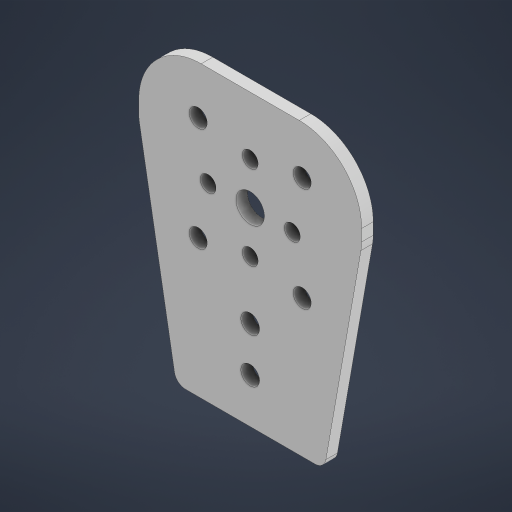
# Autodesk Inventor part: Arm Plate3
Saved by Autodesk Inventor 2024 (Build 280153000, 153)
## iProperties
Created: 2023-10-19
Part Number: Arm Plate3
Material: Generic
Document SubType Name: Modeling
Designer: ellen
Density: 1 g/cm^3
Appearance: Default
Author: ellen
Autodesk Inventor part; units mm, degrees
ref_plane "YZ Plane" through (0, 0, 0) normal (1, 0, 0) x (0, 1, 0)
ref_plane "XZ Plane" through (0, 0, 0) normal (0, 1, 0) x (-1, 0, 0)
ref_plane "XY Plane" through (0, 0, 0) normal (0, 0, 1) x (1, 0, 0)
sketch "Sketch1" plane through (0, 0, 0) normal (0, 0, 1) x (1, 0, 0)
  line L0 (63.5, 76.2) -> (0, 76.2)
  line L1 (0, 76.2) -> (0, 53.975)
  circle A0 centre (31.75, 47.625) radius 4.05
  line L2 (0, 53.975) -> (10.6456, -6.35)
  line L3 (63.5, 53.975) -> (52.8544, -6.35)
  line L4 (10.6456, -6.35) -> (52.8544, -6.35)
  line L5 (63.5, 53.975) -> (63.5, 76.2)
  line L6 (31.75, 76.2) -> (31.75, -6.35)
  circle A1 centre (31.75, 19.05) radius 2.6543
  circle A2 centre (31.75, 6.35) radius 2.6543
  point P0 (0, 0)
  dimension "d0" = 63.5
  dimension "d2" = 8.1
  dimension "d5" = 28.575
  dimension "d50" = 82.55
  dimension "d54" = 5.3086
  dimension "d55" = 57.15
  dimension "d56" = 5.3086
  dimension "d57" = 69.85
  constraints: 14 end point, 3 centre point, 3 point on line, 2 midpoint, 2 parallel, 1 horizontal, 1 perpendicular, 1 vertical
  measures "d0" distance of L0.end L0.start
  measures "d2" diameter of A0
  measures "d5" distance of A0.centre L6.start
  measures "d50" distance between parallel lines of L4 L0
  measures "d54" diameter of A1
  measures "d55" distance from line of L0 A1.centre
  measures "d56" diameter of A2
  measures "d57" distance from line of L0 A2.centre
extrude "Extrusion1" add sketch "Sketch1" along normal blind 3.302 contours L5 L3 L4 L6 A2 A1 A0 L0 | L6 A0 A1 A2 L4 L2 L1 L0
fillet "Fillet9" radius 12.7 1 edges at (63.5, 53.975, 1.651)
fillet "Fillet10" radius 12.7 1 edges at (0, 53.975, 1.651)
fillet "Fillet11" radius 17.78 1 edges at (63.5, 76.2, 1.651)
fillet "Fillet12" radius 17.78 1 edges at (0, 76.2, 1.651)
fillet "Fillet13" radius 3.175 1 edges at (52.8544, -6.35, 1.651)
fillet "Fillet14" radius 3.175 1 edges at (10.6456, -6.35, 1.651)
sketch "Sketch3" plane through (0, 0, 3.302) normal (0, 0, 1) x (1, 0, 0)
  circle A0 centre (31.75, 47.625) radius 4.05 projected
  circle A1 centre (31.75, 47.625) radius 16
  circle A2 centre (31.75, 47.625) radius 8
  circle A3 centre (31.75, 47.625) radius 12
  line L0 (31.75, 47.625) -> (31.75, 69.8383)
  line L1 (31.75, 47.625) -> (53.9633, 47.625) construction
  point P0 (0, 0)
  point P1 (31.75, 59.625)
  dimension "d28" = 24
  dimension "d26" = 32
  dimension "d27" = 16
  dimension "d36" = 90
  constraints: 4 end point, 3 coincident, 2 centre point, 1 horizontal, 1 perpendicular, 1 point on line, 1 vertical alignment, 2 other
  measures "d26" diameter of A1
  measures "d27" diameter of A2
  measures "d36" angle of L1 L0
hole "Hole1" at (31.75, 59.625, 3.302) direction (0, 0, -1) diameter 4.4958 depth 14.1986 tip angle 118 clearance for "Flat Head Machine Screw" size "M4" standard "Ansi Metric M Profile"
pattern_circular "Circular Pattern1" count 4 over 360 about axis through (31.75, 47.625, 0) along (0, 0, 1) of "Hole1"
sketch "Sketch4" plane through (0, 0, 3.302) normal (0, 0, 1) x (1, 0, 0)
  circle A0 centre (31.75, 47.625) radius 4.05 projected
  circle A1 centre (31.75, 47.625) radius 12
  circle A2 centre (31.75, 47.625) radius 16
  circle A3 centre (31.75, 47.625) radius 20.955
  line L0 (45.72, 76.2) -> (17.78, 76.2) projected
  line L1 (31.75, 47.625) -> (51.1677, 67.0427)
  line L2 (31.75, 47.625) -> (59.2107, 47.625) construction
  point P0 (0, 0)
  point P1 (46.5674, 62.4424)
  dimension "d42" = 41.91
  dimension "d40" = 24
  dimension "d41" = 32
  dimension "d58" = 45
  constraints: 4 end point, 3 coincident, 2 centre point, 1 equal length, 1 horizontal, 1 point on line, 3 other
  measures "d40" diameter of A1
  measures "d41" diameter of A2
  measures "d58" angle of L2 L1
hole "Hole2" at (46.5674, 62.4424, 3.302) direction (0, 0, -1) diameter 5.1054 depth 16.256 tip angle 118 clearance for "Flat Head Machine Screw (82)" size "#10" standard "Ansi Unified Screw Threads"
pattern_circular "Circular Pattern2" count 4 over 360 about axis through (31.75, 47.625, 0) along (0, 0, 1) of "Hole2"
equation "\"d54\" = d3"
equation "\"d3\" = 5.3086"
body "Solid1"
